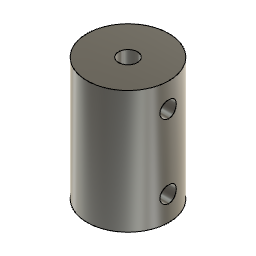
coupling (Autodesk Fusion 360 design; units mm, degrees)
Autodesk Fusion 360 part; units mm, degrees
sketch "Sketch1" plane through (0, 0, 0) normal (0, 0, 1) x (1, 0, 0)
  circle A0 centre (0, 0) radius 5
  dimension "d1" = 10
  constraint coincident A0.centre origin
  measures "d1" diameter of A0
extrude "Extrude1" add sketch "Sketch1" along normal blind 15
sketch "Sketch3" plane through (0, 0, 0) normal (1, 0, 0) x (0, 1, 0)
  line L0 (0, 15) -> (0, 12) construction
  line L1 (0, 0) -> (0, 3) construction
  circle A0 centre (0, 12) radius 1
  circle A1 centre (0, 3) radius 1
  dimension "d5" = 2
  dimension "d6" = 2
  dimension "d9" = 3
  dimension "d10" = 3
  constraint vertical L0
  constraint coincident L1.start origin
  constraint vertical L1
  constraint coincident L0.end A0.centre
  constraint coincident L1.end A1.centre
  measures "d5" diameter of A0
  measures "d6" diameter of A1
  measures "d9" distance of L0.start L0.end
  measures "d10" distance of L1.start L1.end
extrude "Extrude2" cut sketch "Sketch3" along normal mid plane 12
sketch "Sketch4" plane through (0, 0, 15) normal (0, 0, 1) x (-1, 0, 0)
  circle A0 centre (0, 0) radius 5
  circle A1 centre (0, 0) radius 1.15
  dimension "d11" = 2.3
  constraint coincident A0.centre A1.centre
  measures "d11" diameter of A1
extrude "Extrude3" cut sketch "Sketch4" against normal blind 15 contours A1
